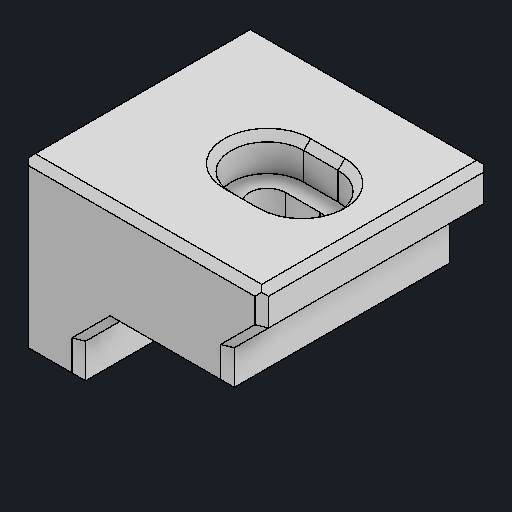
# Autodesk Inventor part: Part1
Saved by Autodesk Inventor 2026.2 (Build 302298000, 298)
## iProperties
Created: 2026-07-19
Part Number: Part1
Material: Generic
Document SubType Name: Modeling
Designer: JoshuaEah
Density: 1 g/cm^3
Appearance: Default
Author: JoshuaEah
Autodesk Inventor part; units mm, degrees
ref_plane "YZ Plane" through (0, 0, 0) normal (1, 0, 0) x (0, 1, 0)
ref_plane "XZ Plane" through (0, 0, 0) normal (0, 1, 0) x (-1, 0, 0)
ref_plane "XY Plane" through (0, 0, 0) normal (0, 0, 1) x (1, 0, 0)
sketch "Sketch1" plane through (0, 0, 0) normal (0, 0, 1) x (1, 0, 0)
  line L0 (0, 0) -> (5, 0)
  line L1 (5, 0) -> (5, 3)
  line L2 (5, 3) -> (8, 6)
  line L3 (8, 6) -> (18, 6)
  line L4 (21, 15) -> (0, 15)
  line L5 (0, 15) -> (0, 0)
  line L6 (18, 6) -> (18, 9)
  line L7 (18, 9) -> (21, 12)
  line L8 (21, 12) -> (21, 15)
  dimension "d0" = 45
  dimension "d2" = 5
  dimension "d4" = 10
  dimension "d6" = 3
  dimension "d7" = 3
  dimension "d8" = 3
  dimension "d25" = 3
  constraints: 18 end point, 3 parallel, 2 perpendicular, 2 vertical, 1 coincident, 1 horizontal
  measures "d0" angle of L2 L1
  measures "d2" distance between parallel lines of L1 L5
  measures "d4" distance of L2.end L3.end
  measures "d6" horizontal distance of L1.end L2.end
  measures "d7" distance of L0.end L1.end
  measures "d8" distance of L3.end L6.end
  measures "d25" distance of L7.end L4.start
extrude "Extrusion1" add sketch "Sketch1" along normal blind 20
sketch "Sketch2" plane through (0, 15, 0) normal (0, 1, 0) x (1, 0, 0)
  line L0 (9.9, -10) -> (16.1, -10) construction
  line L1 (11.5, -11.6) -> (14.5, -11.6)
  line L2 (14.5, -8.4) -> (11.5, -8.4)
  arc A0 (11.5, -8.4) -> (11.5, -11.6) centre (11.5, -10) ccw
  arc A1 (14.5, -11.6) -> (14.5, -8.4) centre (14.5, -10) ccw
  line L3 (11.5, -10) -> (14.5, -10) construction
  line L4 (11.5, -13.175) -> (14.5, -13.175)
  line L5 (14.5, -6.825) -> (11.5, -6.825)
  arc A2 (11.5, -6.825) -> (11.5, -13.175) centre (11.5, -10) ccw
  arc A3 (14.5, -13.175) -> (14.5, -6.825) centre (14.5, -10) ccw
  line L6 (8, 0) -> (18, 0) construction
  line L7 (18, 0) -> (18, -20) construction
  line L8 (8, -20) -> (18, -20) construction
  line L9 (8, 0) -> (8, -20) construction
  point P0 (13, -10)
  point P1 (8.325, -10)
  point P2 (13, -20)
  point P3 (8, -10)
  dimension "d11" = 3.2
  dimension "d16" = 6.35
  dimension "d24" = 3
  constraints: 16 end point, 13 point on circle, 8 tangent, 4 centre point, 4 midpoint, 3 point on line, 2 parallel, 1 coincident, 1 horizontal, 1 horizontal alignment, 1 vertical alignment
  measures "d11" diameter of A1
  measures "d16" diameter of A3
  measures "d24" distance of L3.end A0.centre
extrude "Extrusion2" cut sketch "Sketch2" against normal through all contours A0 L2 A1 L1
extrude "Extrusion3" cut sketch "Sketch2" against normal blind 3 contours A0 L2 A1 L1 | A2 L5 A3 L4
sketch "Sketch3" plane through (0, 0, 0) normal (-1, 0, 0) x (0, 0, 1)
  line L0 (0, 15) -> (0, 0) construction
  line L1 (0, 0) -> (20, 0) construction
  line L2 (20, 15) -> (20, 0) construction
  line L3 (0, 15) -> (20, 15) construction
  line L4 (17, 12) -> (17, 3)
  line L5 (17, 3) -> (3, 3)
  line L6 (3, 3) -> (3, 12)
  line L7 (3, 12) -> (17, 12)
  dimension "d26" = 3
  constraints: 8 end point, 3 other
  measures "d26" distance between parallel lines of L3 L7
extrude "Extrusion4" cut sketch "Sketch3" against normal blind 1
chamfer "Chamfer1" distance 0.6 angle 45 25 edges at (10.5, 15, 20) (10.5, 15, 0) (0, 15, 10) (0, 7.5, 20) (0, 7.5, 0) (0, 0, 10) (2.5, 0, 20) (2.5, 0, 0) (19.5, 10.5, 20) (18, 7.5, 20) (13, 6, 20) (6.5, 4.5, 20) (5, 1.5, 20) (5, 1.5, 0) (6.5, 4.5, 0) (13, 6, 0) (18, 7.5, 0) (19.5, 10.5, 0) (17.675, 15, 10) (13, 15, 13.175) (8.325, 15, 10) (13, 15, 6.825) (21, 13.5, 20) (21, 13.5, 0) (21, 15, 10)
chamfer "Chamfer2" distance 1 angle 45 4 edges at (0, 7.5, 3) (0, 12, 10) (0, 7.5, 17) (0, 3, 10)
equation "\"d7\" = d6"
equation "\"d8\" = d7"
equation "\"d25\" = d7"
body "Solid1"
